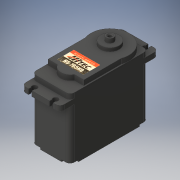
# Autodesk Inventor part: HS-785HB-1111-2017
Saved by Autodesk Inventor 2016 SP2 (Build 200236200, 236)
## iProperties
Created: 2017-02-17
Part Number: HS-785HB-1111-2017
Material: Plastic, Opaque Black
Document SubType Name: Modeling
Designer: 589013
Density: 0.952 g/cm^3
Appearance: Smooth - Dark Gray
Mass: 79.5142 g
Surface Area: 130.905 cm^2
Volume: 83.5234 cm^3
Author: 589013
Autodesk Inventor part; units mm, degrees
ref_plane "YZ Plane" through (0, 0, 0) normal (1, 0, 0) x (0, 1, 0)
ref_plane "XZ Plane" through (0, 0, 0) normal (0, 1, 0) x (-1, 0, 0)
ref_plane "XY Plane" through (0, 0, 0) normal (0, 0, 1) x (1, 0, 0)
sketch "Sketch1" plane through (0, 0, 0) normal (0, 1, 0) x (-1, 0, 0)
  line L0 (-11.1125, 29.21) -> (11.1125, 29.21)
  line L1 (14.2875, 26.035) -> (14.2875, -26.035)
  line L2 (11.1125, -29.21) -> (-11.1125, -29.21)
  line L3 (-14.2875, -26.035) -> (-14.2875, 26.035)
  line L4 (-14.2875, 29.21) -> (14.2875, -29.21) construction
  line L5 (14.2875, 29.21) -> (-14.2875, -29.21) construction
  arc A0 (14.2875, 26.035) -> (11.1125, 29.21) centre (11.1125, 26.035) ccw
  arc A1 (-11.1125, 29.21) -> (-14.2875, 26.035) centre (-11.1125, 26.035) ccw
  arc A2 (-14.2875, -26.035) -> (-11.1125, -29.21) centre (-11.1125, -26.035) ccw
  arc A3 (11.1125, -29.21) -> (14.2875, -26.035) centre (11.1125, -26.035) ccw
  point P0 (0, 0)
  dimension "d0" = 28.575
  dimension "d1" = 58.42
  dimension "d2" = 3.175
  constraints: 12 end point, 8 point on circle, 8 point on line, 8 tangent, 4 centre point, 3 equal radius, 2 midpoint, 2 parallel, 1 horizontal, 1 perpendicular
  measures "d0" distance of L4.end L5.end
  measures "d1" distance of L5.start L4.end
  measures "d2" radius of A0
extrude "Extrusion1" add sketch "Sketch1" along normal blind 46.482
ref_plane "Work Plane1" through (0, 42.672, 0) normal (0, 1, 0) x (1, 0, 0)
sketch "Sketch2" plane through (0, 42.672, 0) normal (0, 1, 0) x (1, 0, 0)
  arc A0 (-11.1125, 29.21) -> (-14.2875, 26.035) centre (-11.1125, 26.035) ccw projected
  line L0 (-11.1125, 29.21) -> (11.1125, 29.21) projected
  arc A1 (14.2875, 26.035) -> (11.1125, 29.21) centre (11.1125, 26.035) ccw projected
  line L1 (14.2875, 26.035) -> (14.2875, -26.035) projected
  arc A2 (11.1125, -29.21) -> (14.2875, -26.035) centre (11.1125, -26.035) ccw projected
  line L2 (11.1125, -29.21) -> (-11.1125, -29.21) projected
  arc A3 (-14.2875, -26.035) -> (-11.1125, -29.21) centre (-11.1125, -26.035) ccw projected
  line L3 (-14.2875, -26.035) -> (-14.2875, 26.035) projected
  line L4 (-11.1125, -36.8935) -> (11.1125, -36.8935)
  line L5 (14.2875, -33.7185) -> (14.2875, 33.7185)
  line L6 (11.1125, 36.8935) -> (-6.604, 36.8935)
  line L7 (-14.2875, 33.7185) -> (-14.2875, -33.7185)
  line L8 (-14.2875, -36.8935) -> (14.2875, 36.8935) construction
  line L9 (14.2875, -36.8935) -> (-14.2875, 36.8935) construction
  arc A4 (-11.1125, 36.8935) -> (-14.2875, 33.7185) centre (-11.1125, 33.7185) ccw
  arc A5 (14.2875, 33.7185) -> (11.1125, 36.8935) centre (11.1125, 33.7185) ccw
  arc A6 (11.1125, -36.8935) -> (14.2875, -33.7185) centre (11.1125, -33.7185) ccw
  arc A7 (-14.2875, -33.7185) -> (-11.1125, -36.8935) centre (-11.1125, -33.7185) ccw
  line L10 (-7.874, -33.655) -> (7.874, -33.655) construction
  line L11 (7.874, -33.655) -> (7.874, 33.655) construction
  line L12 (7.874, 33.655) -> (-7.874, 33.655) construction
  line L13 (-7.874, 33.655) -> (-7.874, -33.655) construction
  line L14 (-7.874, -33.655) -> (7.874, 33.655) construction
  line L15 (7.874, -33.655) -> (-7.874, 33.655) construction
  arc A8 (-9.144, 35.0749) -> (-6.604, 35.0749) centre (-7.874, 33.655) ccw
  line L16 (-9.144, 32.385) -> (-6.604, 32.385) construction
  line L17 (-6.604, 32.385) -> (-6.604, 34.925) construction
  line L18 (-6.604, 34.925) -> (-9.144, 34.925) construction
  line L19 (-9.144, 34.925) -> (-9.144, 32.385) construction
  line L20 (-9.144, 32.385) -> (-6.604, 34.925) construction
  line L21 (-6.604, 32.385) -> (-9.144, 34.925) construction
  line L22 (-9.144, 34.925) -> (-6.604, 34.925) construction
  line L23 (-6.604, 34.925) -> (-6.604, 36.8935)
  line L24 (-6.604, 36.8935) -> (-9.144, 36.8935)
  line L25 (-9.144, 36.8935) -> (-9.144, 34.925)
  arc A9 (-6.604, 35.0749) -> (-9.144, 35.0749) centre (-7.874, 33.655) ccw construction
  line L26 (-9.144, 36.8935) -> (-11.1125, 36.8935)
  line L27 (-6.604, 36.8935) -> (-9.144, 36.8935) construction
  arc A10 (6.604, 35.0749) -> (9.144, 35.0749) centre (7.874, 33.655) ccw
  line L28 (6.604, 36.8935) -> (6.604, 34.925)
  line L29 (9.144, 34.925) -> (9.144, 36.8935)
  line L30 (-14.2875, 0) -> (14.2875, 0) construction
  arc A11 (-6.604, -35.0749) -> (-9.144, -35.0749) centre (-7.874, -33.655) ccw
  line L31 (-6.604, -34.925) -> (-6.604, -36.8935)
  line L32 (-9.144, -36.8935) -> (-9.144, -34.925)
  arc A12 (9.144, -35.0749) -> (6.604, -35.0749) centre (7.874, -33.655) ccw
  line L33 (6.604, -36.8935) -> (6.604, -34.925)
  line L34 (9.144, -34.925) -> (9.144, -36.8935)
  line L35 (6.604, 36.8935) -> (9.144, 36.8935) construction
  line L36 (6.604, -36.8935) -> (9.144, -36.8935) construction
  line L37 (-9.144, -36.8935) -> (-6.604, -36.8935) construction
  line L38 (6.604, 36.8935) -> (9.144, 36.8935)
  line L39 (6.604, -36.8935) -> (9.144, -36.8935)
  line L40 (-9.144, -36.8935) -> (-6.604, -36.8935)
  point P0 (0, 0)
  dimension "d6" = 73.787
  dimension "d7" = 3.175
  dimension "d10" = 15.748
  dimension "d11" = 67.31
  dimension "d12" = 3.81
  dimension "d16" = 2.54
  dimension "d17" = 2.54
  dimension "d20" = 15.748
  constraints: 74 end point, 18 point on circle, 16 point on line, 14 symmetric about line, 12 tangent, 11 parallel, 9 centre point, 8 midpoint, 6 perpendicular, 5 collinear, 4 horizontal, 3 equal radius, 1 coincident, 12 other
  measures "d6" distance of L8.end L9.start
  measures "d7" radius of A4
  measures "d10" distance of L12.end L11.end
  measures "d11" distance of L10.end L11.end
  measures "d12" diameter of A8
  measures "d16" distance of L18.end L17.end
  measures "d17" distance of L17.end L16.end
  measures "d20" distance of A8.centre A10.centre
extrude "Extrusion2" add sketch "Sketch2" against normal blind 3.81 contours A0 L7 A4 L26 L25 A8 L23 L6 L28 A10 L29 A5 L5 A1 L0 | A3 L2 A2 L5 A6 L4 L34 A12 L33 L31 A11 L32 A7 L7 | L24 L23 A8 L25 | L32 A11 L31 L4 | L29 A10 L28 L6 | L4 L33 A12 L34
extrude "Extrusion3" cut sketch "Sketch2" against normal through all contours L24 L23 A8 L25 | L32 A11 L31 L4 | L29 A10 L28 L6 | L4 L33 A12 L34
sketch "Sketch3" plane through (0, 46.482, 0) normal (0, 1, 0) x (1, 0, 0)
  line L0 (-14.2875, 26.035) -> (-14.2875, -26.035) construction
  arc A0 (-14.2875, -26.035) -> (-11.1125, -29.21) centre (-11.1125, -26.035) ccw construction
  line L1 (-11.1125, -29.21) -> (11.1125, -29.21) construction
  arc A1 (11.1125, -29.21) -> (14.2875, -26.035) centre (11.1125, -26.035) ccw construction
  line L2 (14.2875, -26.035) -> (14.2875, 26.035) construction
  arc A2 (14.2875, 26.035) -> (11.1125, 29.21) centre (11.1125, 26.035) ccw construction
  line L3 (11.1125, 29.21) -> (-11.1125, 29.21) construction
  arc A3 (-11.1125, 29.21) -> (-14.2875, 26.035) centre (-11.1125, 26.035) ccw construction
  circle A4 centre (0, 14.9225) radius 14.2875
  line L4 (-13.3985, -18.034) -> (-13.3985, 9.9614)
  line L5 (13.3985, -18.034) -> (13.3985, 9.9614)
  line L6 (-13.3985, -18.034) -> (13.3985, -18.034)
  circle A5 centre (0, -18.034) radius 6.35 construction
  line L7 (0, -18.034) -> (0, -21.844) construction
  arc A6 (-6.35, -18.034) -> (6.35, -18.034) centre (0, -14.6473) ccw
  point P0 (0, 0)
  dimension "d27" = 0.889
  dimension "d28" = 0.889
  dimension "d29" = 47.244
  dimension "d30" = 12.7
  dimension "d31" = 3.81
  constraints: 8 end point, 7 point on circle, 3 centre point, 3 tangent, 3 vertical, 2 point on line, 1 horizontal, 1 midpoint
  measures "d27" distance between parallel lines of L2 L5
  measures "d28" distance between parallel lines of L0 L4
  measures "d29" distance between parallel lines of L3 L6
  measures "d30" diameter of A5
  measures "d31" distance of L7.start L7.end
extrude "Extrusion4" add sketch "Sketch3" along normal blind 3.81
sketch "Sketch4" plane through (0, 50.292, 0) normal (0, 1, 0) x (1, 0, 0)
  arc A0 (13.3985, 9.9614) -> (-13.3985, 9.9614) centre (0, 14.9225) ccw construction
  circle A1 centre (0, 14.9225) radius 6.9215
  point P0 (0, 0)
  dimension "d34" = 13.843
  constraints: 1 centre point, 1 coincident
  measures "d34" diameter of A1
extrude "Extrusion5" add sketch "Sketch4" along normal blind 2.54
sketch "Sketch5" plane through (0, 50.292, 0) normal (0, 1, 0) x (1, 0, 0)
  circle A0 centre (0, 14.9225) radius 6.9215 construction
  arc A1 (-6.35, -18.034) -> (6.35, -18.034) centre (0, -14.6473) ccw construction
  line L0 (6.35, -18.034) -> (13.3985, -18.034) construction
  line L1 (13.3985, -18.034) -> (13.3985, 9.9614) construction
  arc A2 (13.3985, 9.9614) -> (-13.3985, 9.9614) centre (0, 14.9225) ccw construction
  line L2 (-13.3985, 9.9614) -> (-13.3985, -18.034) construction
  line L3 (-13.3985, -18.034) -> (-6.35, -18.034) construction
  line L4 (-9.906, -2.159) -> (9.9036, -2.159) construction
  line L5 (9.9036, -2.159) -> (9.9036, -14.859) construction
  line L6 (9.9036, -14.859) -> (-9.906, -14.859) construction
  line L7 (-9.906, -14.859) -> (-9.906, -2.159) construction
  point P0 (0, 0)
  dimension "d53" = 12.7
  dimension "d59" = 3.175
  dimension "d60" = 3.4925
  dimension "d61" = 3.4949
  constraints: 2 other
  measures "d53" distance of L4.end L5.end
  measures "d59" distance between parallel lines of L6 L0
  measures "d60" distance between parallel lines of L2 L7
  measures "d61" distance between parallel lines of L1 L5
decal "Decal1"
sketch "Sketch6" plane through (0, 52.832, -14.9225) normal (0, 1, 0) x (1, 0, 0)
  circle A0 centre (0, 0) radius 6.9215 construction
  circle A1 centre (0, 0) radius 2.8575
  point P0 (0, -14.9225)
  dimension "d62" = 5.715
  constraints: 1 centre point, 1 coincident
  measures "d62" diameter of A1
extrude "Extrusion6" add sketch "Sketch6" along normal blind 3.175
hole "Hole1" at (0, 56.007, -14.9225) direction (0, -1, 0) diameter 2.54 depth 25.4 tip angle 118 countersink diameter 3.81 countersink angle 82
sketch "Sketch7" plane through (0, 0, 0) normal (0, -1, 0) x (1, 0, 0)
  line L0 (-14.2875, 26.035) -> (-14.2875, -26.035) construction
  arc A0 (-14.2875, -26.035) -> (-11.1125, -29.21) centre (-11.1125, -26.035) ccw construction
  line L1 (-11.1125, -29.21) -> (11.1125, -29.21) construction
  arc A1 (11.1125, -29.21) -> (14.2875, -26.035) centre (11.1125, -26.035) ccw construction
  line L2 (14.2875, -26.035) -> (14.2875, 26.035) construction
  arc A2 (14.2875, 26.035) -> (11.1125, 29.21) centre (11.1125, 26.035) ccw construction
  line L3 (11.1125, 29.21) -> (-11.1125, 29.21) construction
  arc A3 (-11.1125, 29.21) -> (-14.2875, 26.035) centre (-11.1125, 26.035) ccw construction
  line L4 (-14.2875, 26.035) -> (-14.2875, 33.7185) construction
  line L5 (14.2875, -26.035) -> (14.2875, -33.7185) construction
  line L6 (-14.2875, 29.21) -> (14.2875, 29.21) construction
  line L7 (14.2875, 29.21) -> (14.2875, -29.21) construction
  line L8 (14.2875, -29.21) -> (-14.2875, -29.21) construction
  line L9 (-14.2875, -29.21) -> (-14.2875, 29.21) construction
  line L10 (-11.1125, 22.86) -> (-14.2875, 22.86)
  line L11 (-14.2875, 22.86) -> (-14.2875, 29.21)
  line L12 (-14.2875, 29.21) -> (-7.9375, 29.21)
  line L13 (-7.9375, 29.21) -> (-7.9375, 26.035)
  line L14 (-7.9375, 22.86) -> (-14.2875, 29.21) construction
  line L15 (-14.2875, 22.86) -> (-7.9375, 29.21) construction
  line L16 (11.1125, 22.86) -> (14.2875, 22.86)
  line L17 (14.2875, 22.86) -> (14.2875, 29.21)
  line L18 (14.2875, 29.21) -> (7.9375, 29.21)
  line L19 (7.9375, 29.21) -> (7.9375, 26.035)
  line L20 (7.9375, 22.86) -> (14.2875, 29.21) construction
  line L21 (14.2875, 22.86) -> (7.9375, 29.21) construction
  line L22 (-11.1125, -22.86) -> (-14.2875, -22.86)
  line L23 (-14.2875, -22.86) -> (-14.2875, -29.21)
  line L24 (-14.2875, -29.21) -> (-7.9375, -29.21)
  line L25 (-7.9375, -29.21) -> (-7.9375, -26.035)
  line L26 (-7.9375, -22.86) -> (-14.2875, -29.21) construction
  line L27 (-14.2875, -22.86) -> (-7.9375, -29.21) construction
  line L28 (11.1125, -22.86) -> (14.2875, -22.86)
  line L29 (14.2875, -22.86) -> (14.2875, -29.21)
  line L30 (14.2875, -29.21) -> (7.9375, -29.21)
  line L31 (7.9375, -29.21) -> (7.9375, -26.035)
  line L32 (7.9375, -22.86) -> (14.2875, -29.21) construction
  line L33 (14.2875, -22.86) -> (7.9375, -29.21) construction
  arc A4 (-11.1125, 22.86) -> (-7.9375, 26.035) centre (-11.1125, 26.035) ccw
  arc A5 (7.9375, 26.035) -> (11.1125, 22.86) centre (11.1125, 26.035) ccw
  arc A6 (-7.9375, -26.035) -> (-11.1125, -22.86) centre (-11.1125, -26.035) ccw
  arc A7 (11.1125, -22.86) -> (7.9375, -26.035) centre (11.1125, -26.035) ccw
  point P0 (0, 0)
  dimension "d76" = 3.175
  constraints: 56 end point, 10 parallel, 10 point on line, 8 midpoint, 8 point on circle, 8 tangent, 5 horizontal, 5 perpendicular, 4 centre point, 3 equal radius
  measures "d76" radius of A4
extrude "Extrusion7" cut sketch "Sketch7" against normal blind 1.27
body "Solid1"
